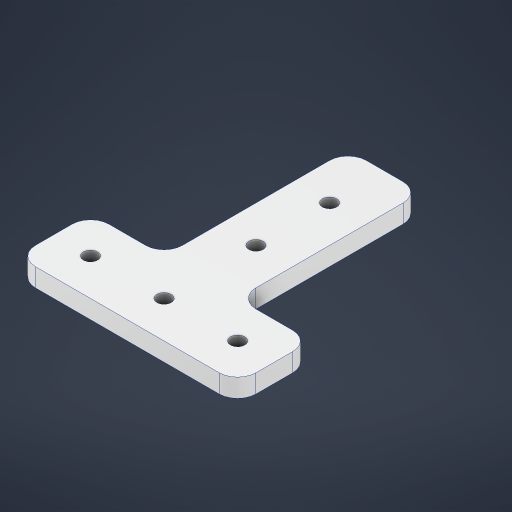
# Autodesk Inventor part: STRU_020_DVBSBracket1
Saved by Autodesk Inventor 2024.2 (Build 282272000, 272)
## iProperties
Created: 2024-07-28
Part Number: STRU_020_DVBSBracket1
Material: Aluminum 6061
Document SubType Name: Modeling
Designer: Bryan
Density: 2.7 g/cm^3
Appearance: Aluminum - Flat
Author: Bryan
Autodesk Inventor part; units mm, degrees
ref_plane "YZ Plane" through (0, 0, 0) normal (1, 0, 0) x (0, 1, 0)
ref_plane "XZ Plane" through (0, 0, 0) normal (0, 1, 0) x (-1, 0, 0)
ref_plane "XY Plane" through (0, 0, 0) normal (0, 0, 1) x (1, 0, 0)
sketch "Sketch1" plane through (0, 0, 0) normal (0, 1, 0) x (-1, 0, 0)
  line L0 (-38.1, 0) -> (38.1, 0)
  line L1 (38.1, 0) -> (38.1, -25.4)
  line L2 (38.1, -25.4) -> (12.7, -25.4)
  line L3 (12.7, -25.4) -> (12.7, -88.9)
  line L4 (12.7, -88.9) -> (-12.7, -88.9)
  line L5 (-12.7, -88.9) -> (-12.7, -25.4)
  line L6 (-12.7, -25.4) -> (-38.1, -25.4)
  line L7 (-38.1, -25.4) -> (-38.1, 0)
  circle A0 centre (0, -12.7) radius 2.4892
  circle A1 centre (25.4, -12.7) radius 2.4892
  line L8 (0, 0) -> (0, -88.9) construction
  circle A2 centre (-25.4, -12.7) radius 2.4892
  circle A3 centre (0, -44.45) radius 2.4892
  circle A4 centre (0, -69.85) radius 2.4892
  point P0 (38.1, -12.7)
  point P1 (0, -44.45)
  dimension "d0" = 76.2
  dimension "d1" = 25.4
  dimension "d2" = 25.4
  dimension "d3" = 63.5
  dimension "d4" = 4.9784
  dimension "d5" = 25.4
  dimension "d6" = 31.75
  dimension "d7" = 25.4
  constraints: 18 end point, 5 centre point, 5 midpoint, 3 equal radius, 3 point on line, 3 vertical, 2 equal length, 2 horizontal, 2 horizontal alignment, 1 coincident, 1 perpendicular, 1 symmetric about line, 1 vertical alignment, 1 other
  measures "d0" distance of L0.start L0.end
  measures "d1" distance of L0.end L1.end
  measures "d2" distance of L3.end L4.end
  measures "d3" distance from line of L2.end L4
  measures "d4" diameter of A0
  measures "d5" distance of A0.centre A1.centre
  measures "d6" distance of A3.centre A0.centre
  measures "d7" distance of A4.centre point (0, -44.45)
extrude "Extrusion1" add sketch "Sketch1" along normal blind 6.35
fillet "Fillet1" radius 6.35 8 edges at (-38.1, 3.175, 0) (-38.1, 3.175, -25.4) (-12.7, 3.175, -25.4) (-12.7, 3.175, -88.9) (12.7, 3.175, -88.9) (12.7, 3.175, -25.4) (38.1, 3.175, -25.4) (38.1, 3.175, 0)
body "Solid1"
